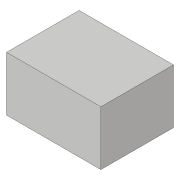
# Autodesk Inventor part: rectangle_1
Saved by Autodesk Inventor 2022 Beta2 (Build 260130000, 130) ContinuousBuild 0
## iProperties
Created: 2018-02-02
Part Number: rectangle_1
Material: Generic
Document SubType Name: Modeling
Designer: jmacmillan
Density: 1 g/cm^3
Appearance: Default
Author: jmacmillan
Autodesk Inventor part; units mm, degrees
ref_plane "YZ Plane" through (0, 0, 0) normal (1, 0, 0) x (0, 1, 0)
ref_plane "XZ Plane" through (0, 0, 0) normal (0, 1, 0) x (-1, 0, 0)
ref_plane "XY Plane" through (0, 0, 0) normal (0, 0, 1) x (1, 0, 0)
sketch "Sketch1" plane through (0, 0, 0) normal (0, 1, 0) x (-1, 0, 0)
  line L0 (13, 10) -> (-13, 10)
  line L1 (-13, 10) -> (-13, -10)
  line L2 (-13, -10) -> (13, -10)
  line L3 (13, -10) -> (13, 10)
  line L4 (0, -14) -> (0, 14) projected
  line L5 (-18.2, 0) -> (18.2, 0) projected
  point P0 (0, 0)
  dimension "d0" = 26
  dimension "d1" = 20
  constraints: 8 end point, 2 equal length, 1 horizontal, 1 perpendicular, 2 other
  measures "d0" distance of L1.end L2.end
  measures "d1" distance of L2.end L0.start
extrude "Extrusion1" add sketch "Sketch1" along normal mid plane 15
body "Solid1"
